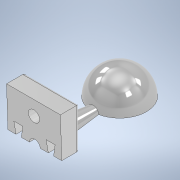
# Autodesk Inventor part: markerWithRodEnd
Saved by Autodesk Inventor 2022 (Build 260153000, 153)
## iProperties
Created: 2021-09-13
Part Number: markerWithRodEnd
Material: ABS Plastic
Document SubType Name: Modeling
Designer: tecware
Density: 1.06 g/cm^3
Appearance: Aluminum - Polished
Author: tecware
## iProperties of the stored document markerWithRodEnd_3DPrint.ipt
Created: 2021-09-13
Part Number: markerWithRodEnd_3DPrint
Material: Generic
Document SubType Name: Modeling
Designer: tecware
Density: 1 g/cm^3
Appearance: Default
Author: tecware
Autodesk Inventor part; units mm, degrees
ref_plane "YZ Plane" through (0, 0, 0) normal (1, 0, 0) x (0, 1, 0)
ref_plane "XZ Plane" through (0, 0, 0) normal (0, 1, 0) x (-1, 0, 0)
ref_plane "XY Plane" through (0, 0, 0) normal (0, 0, 1) x (1, 0, 0)
sketch "Sketch1" plane through (0, 0, 0) normal (0, 1, 0) x (-1, 0, 0)
  line L0 (0, 0) -> (-2, 0)
  line L1 (-2, 0) -> (-4, 0)
  line L2 (0, 0) -> (0, -15)
  line L3 (0, -15) -> (0, -25)
  circle A0 centre (0, -25) radius 10
  line L4 (-1.5, -15.1131) -> (0, -15.1131)
  line L5 (0, -15.1131) -> (0, -15)
  line L6 (-1.5, -15) -> (-1.5, -15.1131)
  line L7 (-1.5, -15.1131) -> (-2, 0)
  line L8 (0, -15) -> (-1.5, -15)
  line L9 (-1.5, -15) -> (-2, -15)
  line L10 (-2, -15) -> (-2, -15.202)
  line L11 (-2, -15.202) -> (-4, 0)
  line L12 (0, -25) -> (0, -35)
  circle A1 centre (0, -25) radius 9.2
  line L13 (-1.5, -15.1131) -> (-1.4733, -15.9187)
  point P0 (0, -34.2)
  dimension "d7" = 18.4
  dimension "d2" = 15
  dimension "d4" = 10
  dimension "d6" = 0.5
  dimension "d10" = 1.5
  dimension "d11" = 2
  dimension "d12" = 2
  constraints: 28 end point, 4 point on circle, 3 perpendicular, 3 point on line, 2 coincident, 2 horizontal, 2 vertical, 1 centre point, 1 parallel, 1 tangent, 3 other
  measures "d2" distance of L0.start L2.end
  measures "d4" distance of L2.end L3.end
  measures "d6" distance of L6.start L9.end
  measures "d10" distance of L4.start L4.end
  measures "d11" distance of L0.start L0.end
  measures "d12" distance of L0.end L1.end
revolve "Revolution1" add sketch "Sketch1" angle 180 about axis through (0, 0, 0) along (0, 0, 1) contours L7 L9 L10 L11 L1 | L7 A0 L10 L9 | L13 A1 L12 A0
sketch "Sketch2" plane through (0, 0, 0) normal (0, 0, 1) x (1, 0, 0)
  line L0 (5, 0) -> (-5, 0)
  line L1 (-14, 0) -> (14, 0) projected
  arc A0 (2, 0) -> (-2, 0) centre (0, 0) ccw projected
  line L2 (0, 0) -> (0, 16) construction
  line L3 (-10, 0) -> (10, 0)
  line L4 (10, 0) -> (10, 15)
  line L5 (10, 15) -> (-10, 15)
  line L6 (-10, 15) -> (-10, 0)
  point P0 (0, 0)
  point P1 (0, 0)
  point P2 (-10, 0)
  point P3 (10, 0)
  dimension "d29" = 20
  dimension "d33" = 15
  dimension "d34" = 15
  constraints: 12 end point, 2 midpoint, 2 parallel, 1 collinear, 1 horizontal, 1 perpendicular
  measures "d29" distance of L4.end L5.end
  measures "d33" distance between parallel lines of L1 L5
  measures "d34" distance of L5.end L3.start
extrude "Base" add sketch "Sketch2" along normal blind 7 contours L0 A0 L1 L6 L5 L4
sketch "Sketch3" plane through (0, 0, 0) normal (0, 0, -1) x (-1, 0, 0)
  line L0 (0, -3) -> (0, 18) projected
  line L1 (-10, 15) -> (10, 15) projected
  point P0 (0, 0)
  point P1 (0, 9.5)
  dimension "d30" = 5.5
  constraints: 1 point on line
  measures "d30" distance from line of L1 point (0, 9.5)
hole "Screw Hole" at (0, 9.5, 0) direction (0, 0, 1) diameter 4.2 end through all counterbore diameter 8 counterbore depth 3
sketch "Sketch4" plane through (0, 0, 0) normal (0, 0, -1) x (-1, 0, 0)
  line L0 (-2, 0) -> (-10, 0) projected
  line L1 (0, 0) -> (0, -2) construction
  line L2 (6, 0) -> (6, 6)
  line L3 (6, 6) -> (8, 6)
  line L4 (6, 6) -> (4, 6)
  line L5 (4, 6) -> (5, 0)
  line L6 (7, 0) -> (8, 6)
  line L7 (7, 0) -> (5, 0)
  line L8 (10, 0) -> (2, 0) projected
  line L9 (6, 0) -> (6, 4)
  line L10 (7.6667, 4) -> (4.3333, 4)
  line L11 (0, 0) -> (0, 18)
  line L12 (10, 0) -> (4, 0) projected
  line L13 (-6, 0) -> (-6, 6)
  line L14 (-6, 6) -> (-8, 6)
  line L15 (-6, 6) -> (-4, 6)
  line L16 (-4, 6) -> (-5, 0)
  line L17 (-7, 0) -> (-8, 6)
  line L18 (-7, 0) -> (-5, 0)
  line L19 (-6, 0) -> (-6, 4)
  line L20 (-7.6667, 4) -> (-4.3333, 4)
  point P0 (5, 0)
  point P1 (-5, 0)
  point P2 (-5, 0)
  constraints: 36 end point, 12 symmetric about line, 7 point on line, 1 collinear, 1 midpoint, 1 perpendicular, 1 vertical
extrude "Keyway" cut sketch "Sketch4" against normal through all contours L0 L13 L20 L16 | L0 L17 L20 L13 | L7 L5 L10 L2 | L2 L10 L6 L7
sketch "Sketch5" plane through (10, 0, 0) normal (1, 0, 0) x (0, 0, -1)
  line L0 (0, 15) -> (-7, 15) projected
  line L1 (0, 15) -> (-7, 15) projected
  line L2 (0, 0) -> (-7, 0) projected
  line L3 (-7, 15) -> (-7, 0) projected
  line L4 (-7, 15) -> (-7, 0)
  line L5 (-7, 0) -> (-6.5, 0)
  line L6 (-7, 15) -> (-6.5, 0)
  dimension "d37" = 0.5
  constraints: 6 end point, 1 perpendicular, 1 point on line
  measures "d37" distance of L2.end L5.end
extrude "Taper" cut sketch "Sketch5" against normal through all
fillet "Fillet1" radius 1 3 edges at (-10, 7.5, 0) (0, 15, 0) (10, 7.5, 0)
equation "\"d34\" = d33"
body "Solid1"
